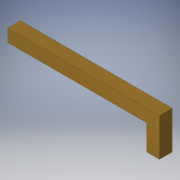
# Autodesk Inventor part: IRIOPin
Saved by Autodesk Inventor 2018 (Build 220112000, 112)
## iProperties
Created: 2018-01-13
Part Number: IRIOPin
Material: Brass, Soft Yellow
Document SubType Name: Modeling
Designer: Kyle-HP
Density: 8.47 g/cm^3
Appearance: Brass - Satin
Author: Kyle-HP
Autodesk Inventor part; units mm, degrees
ref_plane "YZ Plane" through (0, 0, 0) normal (1, 0, 0) x (0, 1, 0)
ref_plane "XZ Plane" through (0, 0, 0) normal (0, 1, 0) x (-1, 0, 0)
ref_plane "XY Plane" through (0, 0, 0) normal (0, 0, 1) x (1, 0, 0)
sketch "Sketch1" plane through (0, 0, 0) normal (0, 0, 1) x (1, 0, 0)
  line L0 (0, 0) -> (7.62, 0)
  line L1 (7.62, 0) -> (7.62, -1.905)
  line L2 (7.62, -1.905) -> (6.985, -1.905)
  line L3 (0, 0) -> (0, -0.635)
  line L4 (0, -0.635) -> (6.985, -0.635)
  line L5 (6.985, -0.635) -> (6.985, -1.905)
  dimension "d0" = 7.62
  dimension "d1" = 1.905
  dimension "d2" = 0.635
  dimension "d3" = 0.635
  constraints: 12 end point, 3 horizontal, 2 vertical, 1 perpendicular
  measures "d0" distance of L0.start L0.end
  measures "d1" distance of L0.end L1.end
  measures "d2" distance of L1.end L2.end
  measures "d3" distance of L0.start L3.end
extrude "Extrusion1" add sketch "Sketch1" along normal blind 0.635
body "Solid1"
